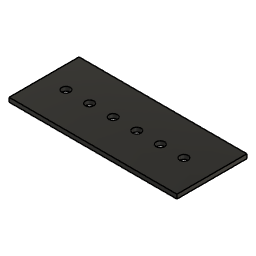
Ensamble v2 (Autodesk Fusion 360 archive; units mm, degrees)
design "Base"
Autodesk Fusion 360 part; units mm, degrees
sketch "Boceto1" plane through (0, 0, 0) normal (0, 0, 1) x (1, 0, 0)
  line L0 (0, 0) -> (120, 0)
  line L1 (120, 0) -> (120, 50)
  line L2 (120, 50) -> (0, 50)
  line L3 (0, 50) -> (0, 0)
  dimension "d1" = 120
  dimension "d2" = 50
  constraint horizontal L0
  constraint vertical L1
  constraint horizontal L2
  constraint vertical L3
  constraint coincident L0.start L3.end
  measures "d1" distance of L0.start L0.end
  measures "d2" distance of L0.start L2.end
extrude "Extruir1" add sketch "Boceto1" along normal blind 3
sketch "Boceto2" plane through (0, 0, 3) normal (0, 0, 1) x (-1, 0, 0)
  line L0 (0, -50) -> (0, 0)
  line L1 (0, 0) -> (-120, 0)
  line L2 (-120, 0) -> (-120, -50)
  line L3 (-120, -50) -> (0, -50)
  line L4 (-120, -25) -> (0, -25)
  line L5 (-120, -25) -> (-100, -25)
  circle A0 centre (-100, -25) radius 3
  line L6 (-100, -25) -> (-83.13, -25)
  circle A1 centre (-83.13, -25) radius 3
  line L7 (-83.13, -25) -> (-66.26, -25)
  circle A2 centre (-66.26, -25) radius 3
  line L8 (-66.26, -25) -> (-49.39, -25)
  circle A3 centre (-49.39, -25) radius 3
  line L9 (-49.39, -25) -> (-32.52, -25)
  circle A4 centre (-32.52, -25) radius 3
  line L10 (-32.52, -25) -> (-15.65, -25)
  circle A5 centre (-15.65, -25) radius 3
  dimension "d5" = 20
  dimension "d6" = 6
  dimension "d7" = 16.87
  dimension "d8" = 6
  dimension "d9" = 16.87
  dimension "d11" = 6
  dimension "d12" = 16.87
  dimension "d13" = 6
  dimension "d14" = 16.87
  dimension "d15" = 6
  dimension "d16" = 16.87
  dimension "d17" = 6
  constraint midpoint L2 L4.start
  constraint midpoint L0 L4.end
  constraint perpendicular L2 L5
  constraint coincident L5.end A0.centre
  constraint parallel L4 L6
  constraint coincident L6.end A1.centre
  constraint parallel L4 L7
  constraint coincident L7.end A2.centre
  constraint parallel L4 L8
  constraint coincident L8.end A3.centre
  constraint parallel L4 L9
  constraint coincident L9.end A4.centre
  constraint coincident L4 L10.end
  constraint coincident L10.end A5.centre
  measures "d5" distance of L4.start L5.end
  measures "d6" diameter of A0
  measures "d7" distance of L5.end L6.end
  measures "d8" diameter of A1
  measures "d9" distance of L6.end L7.end
  measures "d11" diameter of A2
  measures "d12" distance of L7.end L8.end
  measures "d13" diameter of A3
  measures "d14" distance of L8.end L9.end
  measures "d15" diameter of A4
  measures "d16" distance of L9.end L10.end
  measures "d17" diameter of A5
extrude "Extruir2" cut sketch "Boceto2" against normal blind 3 contours L4 L10 A5 | L4 L10 A5 | L4 L5 A0 L6 | L4 L5 A0 L6 | L4 L9 A4 L10 | L4 L9 A4 L10 | L4 L6 A1 L7 | L4 L6 A1 L7 | L4 L8 A3 L9 | L4 L8 A3 L9 | L4 L7 A2 L8 | L4 L7 A2 L8
equation "d6 = D_b"
equation "d7 = Dc"
equation "d8 = D_b"
equation "d9 = Dc"
equation "Dc = 16.87 mm"
equation "d11 = D_b"
equation "d12 = Dc"
equation "d13 = D_b"
equation "d14 = Dc"
equation "d15 = D_b"
equation "d16 = Dc"
equation "d17 = D_b"
equation "D_b = 6 mm"

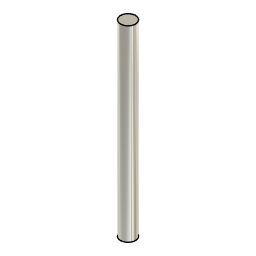
design "Eje"
Autodesk Fusion 360 part; units mm, degrees
sketch "Boceto1" plane through (0, 0, 0) normal (0, 0, 1) x (1, 0, 0)
  circle A0 centre (0, 0) radius 1
  dimension "d1" = 2
  constraint coincident A0.centre origin
  measures "d1" diameter of A0
extrude "Extruir1" add sketch "Boceto1" along normal blind 25
